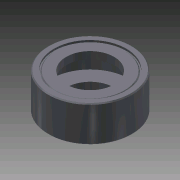
# Autodesk Inventor part: out casing 1764
Saved by Autodesk Inventor 2011 (Build 150239000, 239)
## iProperties
Created: 2009-01-08
Part Number: out casing 1764
Document SubType Name: Modeling
Designer: pmulligan
Density: 1 g/cm^3
Author: pmulligan
Autodesk Inventor part; units mm, degrees
ref_plane "YZ Plane" through (0, 0, 0) normal (1, 0, 0) x (0, 1, 0)
ref_plane "XZ Plane" through (0, 0, 0) normal (0, 1, 0) x (-1, 0, 0)
ref_plane "XY Plane" through (0, 0, 0) normal (0, 0, 1) x (1, 0, 0)
sketch "Sketch1" plane through (0, 0, 0) normal (0, 0, 1) x (1, 0, 0)
  line L0 (-27.5463, 4.2273) -> (-26.0223, 4.2273)
  line L1 (-26.0223, 4.2273) -> (-26.0223, -5.2469)
  line L2 (-26.0223, -5.2469) -> (-27.5463, -5.2469)
  line L3 (-27.5463, -5.2469) -> (-27.5463, 4.2273)
  line L4 (-16.4338, 9.0278) -> (-16.4338, -15.3549)
  dimension "d0" = 9.4742
  dimension "d1" = 1.524
  dimension "d2" = 11.1125
  constraints: 10 end point, 3 parallel, 1 horizontal, 1 perpendicular
  measures "d0" distance of L2.end L0.start
  measures "d1" distance of L0.start L0.end
  measures "d2" distance between parallel lines of L4 L3
revolve "Revolution1" add sketch "Sketch1" angle 360 about axis through (-16.4338, 9.0278, 0) along (0, -1, 0)
ref_plane "Work Plane1" through (-16.4338, 3.9733, 0) normal (0, 1, 0) x (1, 0, 0)
sketch "Sketch2" plane through (-16.4338, 3.9733, 0) normal (0, 1, 0) x (1, 0, 0)
  circle A0 centre (0, 0) radius 11.1125
  circle A1 centre (0, 0) radius 6.35
  dimension "d5" = 12.7
  dimension "d35" = 22.225
  constraints: 2 centre point, 1 coincident
  measures "d5" diameter of A1
  measures "d35" diameter of A0
extrude "Extrusion1" add sketch "Sketch2" against normal blind 1.9207
ref_plane "Work Plane2" through (-16.4338, -4.9929, 0) normal (0, -1, 0) x (1, 0, 0)
sketch "Sketch3" plane through (-16.4338, -4.9929, 0) normal (0, -1, 0) x (1, 0, 0)
  circle A0 centre (0, 0) radius 11.1125
  circle A1 centre (0, 0) radius 6.35
  dimension "d9" = 12.7
  dimension "d34" = 22.225
  constraints: 2 centre point, 1 coincident
  measures "d9" diameter of A1
  measures "d34" diameter of A0
extrude "Extrusion2" add sketch "Sketch3" against normal blind 1.9207
ref_plane "Work Plane3" through (-16.4338, -3.0722, 0) normal (0, 1, 0) x (1, 0, 0)
sketch "Sketch4" plane through (-16.4338, -3.0722, 0) normal (0, 1, 0) x (1, 0, 0)
  circle A0 centre (0, 0) radius 10.3505
  dimension "d13" = 20.701
  constraints: 1 centre point
  measures "d13" diameter of A0
extrude "Extrusion3" cut sketch "Sketch4" along normal blind 5.1248
sketch "Sketch5" plane through (-16.4338, -4.9929, 0) normal (0, -1, 0) x (1, 0, 0)
  circle A0 centre (0, 0) radius 9.5885 projected
  circle A1 centre (0, 0) radius 9.3345
  dimension "d16" = 0.254
  constraints: 1 centre point, 1 coincident
  measures "d16" radial gap between concentric circles of A0 A1
extrude "Extrusion4" cut sketch "Sketch5" against normal blind 0.254
chamfer "Chamfer1" distance 0.254 angle 45 1 edges at (-25.7683, -4.9929, 0)
sketch "Sketch6" plane through (-16.4338, 3.9733, 0) normal (0, 1, 0) x (1, 0, 0)
  circle A0 centre (0, 0) radius 9.5885 projected
  circle A1 centre (0, 0) radius 9.3345
  dimension "d22" = 0.254
  constraints: 1 centre point, 1 coincident
  measures "d22" radial gap between concentric circles of A0 A1
extrude "Extrusion5" cut sketch "Sketch6" against normal blind 0.254
chamfer "Chamfer2" distance 0.254 angle 45 1 edges at (-25.7683, 3.9733, 0)
chamfer "Chamfer3" distance 0.254 angle 45 1 edges at (-5.3213, -5.2469, 0)
chamfer "Chamfer4" distance 0.254 angle 45 1 edges at (-5.3213, 4.2273, 0)
body "Solid1"
